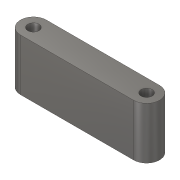
# Autodesk Inventor part: OZZ-CasterRiserBlock
Saved by Autodesk Inventor 2019.4 (Build 234330000, 330)
## iProperties
Created: 2020-02-24
Part Number: OZZ-CasterRiserBlock
Material: Steel, Alloy
Document SubType Name: Modeling
Designer: Lord of Xy
Density: 7.73 g/cm^3
Appearance: Semi-Polished
Author: Lord of Xy
Autodesk Inventor part; units mm, degrees
ref_plane "YZ Plane" through (0, 0, 0) normal (1, 0, 0) x (0, 1, 0)
ref_plane "XZ Plane" through (0, 0, 0) normal (0, 1, 0) x (-1, 0, 0)
ref_plane "XY Plane" through (0, 0, 0) normal (0, 0, 1) x (1, 0, 0)
sketch "Sketch1" plane through (0, 0, 0) normal (0, 1, 0) x (-1, 0, 0)
  line L0 (-27.7812, 0) -> (27.7812, 0) construction
  line L1 (-27.7812, -6.35) -> (27.7812, -6.35)
  line L2 (27.7812, 6.35) -> (-27.7812, 6.35)
  arc A0 (-27.7812, 6.35) -> (-27.7812, -6.35) centre (-27.7812, 0) ccw
  arc A1 (27.7812, -6.35) -> (27.7812, 6.35) centre (27.7812, 0) ccw
  circle A2 centre (27.7812, 0) radius 2.7781
  circle A3 centre (-27.7812, 0) radius 2.7781
  point P0 (0, 0)
  dimension "d0" = 5.5563
  dimension "d1" = 55.5625
  dimension "d2" = 6.35
  constraints: 8 end point, 4 centre point, 4 point on circle, 4 tangent, 2 coincident, 1 equal radius, 1 horizontal, 1 midpoint, 1 parallel
  measures "d0" diameter of A3
  measures "d1" distance of L0.start L0.end
  measures "d2" radius of A1
extrude "Extrusion1" add sketch "Sketch1" along normal blind 25.4
body "Solid1"
